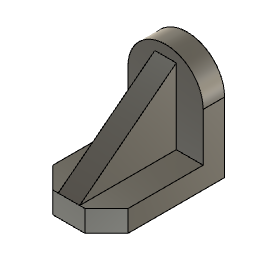
A1 (Autodesk Fusion 360 design; units mm, degrees)
Autodesk Fusion 360 part; units mm, degrees
sketch "Sketch1" plane through (0, 0, 0) normal (0, 0, 1) x (1, 0, 0)
  line L0 (21, -33) -> (-21, -33)
  line L1 (-21, -33) -> (-21, 33)
  line L2 (-21, 33) -> (21, 33)
  line L3 (21, 33) -> (21, -33)
  line L4 (21, -33) -> (-21, 33) construction
  line L5 (-21, -33) -> (21, 33) construction
  dimension "d1" = 42
  dimension "d2" = 66
  constraint horizontal L0
  constraint perpendicular L0 L1
  constraint parallel L0 L2
  constraint parallel L1 L3
  constraint coincident L4 origin
  constraint coincident L5 origin
  measures "d1" distance of L1.end L2.end
  measures "d2" distance of L0.end L1.end
extrude "Extrude1" add sketch "Sketch1" along normal blind 12
sketch "Sketch2" plane through (0, 0, 12) normal (0, 0, 1) x (-1, 0, 0)
  line L0 (-21, -33) -> (21, -33)
  line L1 (21, -33) -> (21, 33)
  line L2 (21, 33) -> (-21, 33)
  line L3 (-21, 33) -> (-21, -33)
  line L4 (-21, -33) -> (21, -33)
  line L5 (21, -33) -> (21, -21)
  line L6 (21, -21) -> (-21, -21)
  line L7 (-21, -21) -> (-21, -33)
  dimension "d5" = 42
  dimension "d6" = 12
  constraint horizontal L4
  constraint vertical L5
  constraint horizontal L6
  constraint vertical L7
  constraint coincident L0.start L3.end
  measures "d5" distance of L0.start L0.end
  measures "d6" distance of L0.start L6.end
extrude "Extrude2" add sketch "Sketch2" along normal blind 48 contours L0 L1 L3 L4 L5 L6 L7
fillet "Fillet1" radius 21 2 edges at (-21, 27, 60) (21, 27, 60)
sketch "Sketch3" plane through (0, 0, 0) normal (1, 0, 0) x (0, 1, 0)
  line L0 (21, 54) -> (21, 12)
  line L1 (21, 12) -> (-33, 12)
  line L2 (-33, 12) -> (21, 54)
  dimension "d11" = 42
  dimension "d12" = 54
  constraint vertical L0
  constraint perpendicular L0 L1
  measures "d11" distance of L0.start L0.end
  measures "d12" distance of L0.end L1.end
extrude "Extrude3" add sketch "Sketch3" along normal mid plane 12
chamfer "Chamfer1" distance 12 angle 45 2 edges at (-21, -33, 6) (21, -33, 6)
equation "d7 = 60 mm - 12 mm"
equation "d12 = 66 mm - 12 mm"
named bodies: "A1"
